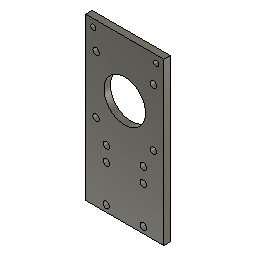
Carriage Plate P3 Printer (Autodesk Fusion 360 design; units mm, degrees)
Autodesk Fusion 360 part; units mm, degrees
sketch "Sketch1" plane through (0, 0, 0) normal (0, 1, 0) x (1, 0, 0)
  line L0 (32, 30) -> (-32, 30)
  line L1 (-32, 30) -> (-32, -30)
  line L2 (-32, -30) -> (32, -30)
  line L3 (32, -30) -> (32, 30)
  line L4 (32, 30) -> (-32, -30) construction
  line L5 (-32, 30) -> (32, -30) construction
  line L6 (-10, 2.5) -> (10, 2.5) construction
  line L7 (10, 2.5) -> (10, 22.5) construction
  line L8 (10, 22.5) -> (-10, 22.5) construction
  line L9 (-10, 22.5) -> (-10, 2.5) construction
  circle A0 centre (-10, 2.5) radius 1.75
  circle A1 centre (10, 2.5) radius 1.75
  circle A2 centre (10, 22.5) radius 1.75
  circle A3 centre (-10, 22.5) radius 1.75
  line L10 (28, 26) -> (-28, 26)
  line L11 (-28, 26) -> (-28, -26)
  line L12 (-28, -26) -> (28, -26)
  line L13 (28, -26) -> (28, 26)
  line L14 (-28, -26) -> (-24, -26)
  line L15 (-24, -26) -> (-24, 0)
  line L16 (-24, 0) -> (-28, 0)
  line L17 (-28, 0) -> (-28, -26)
  line L18 (28, -26) -> (24, -26)
  line L19 (24, -26) -> (24, 0)
  line L20 (24, 0) -> (28, 0)
  line L21 (28, 0) -> (28, -26)
  line L22 (21.15, -30) -> (-21.15, -30) construction
  line L23 (-21.15, -30) -> (-21.15, -22) construction
  line L24 (21.15, -22) -> (21.15, -30) construction
  line L25 (-21.15, -30) -> (21.15, -30)
  line L26 (21.15, -30) -> (21.15, -10)
  line L27 (21.15, -10) -> (-21.15, -10)
  line L28 (-21.15, -10) -> (-21.15, -30)
  line L29 (21.15, -10) -> (-21.15, -10)
  line L30 (-21.15, -10) -> (-21.15, -52.3)
  line L31 (-21.15, -52.3) -> (21.15, -52.3)
  line L32 (21.15, -52.3) -> (21.15, -10)
  line L33 (21.15, -52.3) -> (-21.15, -10) construction
  line L34 (-21.15, -52.3) -> (21.15, -10) construction
  line L35 (-15.5, -15.65) -> (15.5, -15.65) construction
  line L36 (15.5, -15.65) -> (15.5, -46.65) construction
  line L37 (15.5, -46.65) -> (-15.5, -46.65) construction
  line L38 (-15.5, -46.65) -> (-15.5, -15.65) construction
  line L39 (-15.5, -15.65) -> (15.5, -46.65) construction
  line L40 (15.5, -15.65) -> (-15.5, -46.65) construction
  circle A4 centre (15.5, -46.65) radius 1.75
  circle A5 centre (-15.5, -46.65) radius 1.75
  circle A6 centre (-15.5, -15.65) radius 1.75
  circle A7 centre (15.5, -15.65) radius 1.75
  circle A8 centre (0, -31.15) radius 11.25
  line L41 (-21.15, -26) -> (21.15, -26)
  line L42 (21.15, -26) -> (21.15, 26)
  line L43 (21.15, 26) -> (-21.15, 26)
  line L44 (-21.15, 26) -> (-21.15, -26)
  line L45 (21.15, 26) -> (-21.15, 26)
  line L46 (-21.15, 26) -> (-21.15, -1)
  line L47 (-21.15, -1) -> (21.15, -1)
  line L48 (21.15, -1) -> (21.15, 26)
  line L49 (21.15, -1) -> (-21.15, -1) construction
  line L50 (-21.15, -1) -> (-21.15, -10) construction
  line L51 (-21.15, -10) -> (21.15, -10) construction
  line L52 (21.15, -10) -> (21.15, -1) construction
  circle A9 centre (-10, -5.5) radius 1.75
  circle A10 centre (10, -5.5) radius 1.75
  line L53 (21.15, -52.3) -> (-21.15, -52.3)
  line L54 (-21.15, -52.3) -> (-21.15, -61.3)
  line L55 (-21.15, -61.3) -> (21.15, -61.3)
  line L56 (21.15, -61.3) -> (21.15, -52.3)
  circle A11 centre (-17, -57.2801) radius 1.4
  circle A12 centre (17, -57.3) radius 1.4
  point P0 (0, -26)
  point P1 (0, -31.15)
  dimension "d1" = 64
  dimension "d2" = 60
  dimension "d3" = 20
  dimension "d4" = 20
  dimension "d6" = 22
  dimension "d7" = 3.5
  dimension "d8" = 3.5
  dimension "d9" = 3.5
  dimension "d10" = 3.5
  dimension "d11" = -4
  dimension "d12" = 4
  dimension "d13" = 4
  dimension "d40" = 3.5
  dimension "d41" = 26
  dimension "d42" = 26
  dimension "d43" = 42.3
  dimension "d44" = 8
  dimension "d45" = 20
  dimension "d46" = 42.3
  dimension "d49" = 31
  dimension "d50" = 31
  dimension "d51" = 3.5
  dimension "d52" = 3.5
  dimension "d53" = 3.5
  dimension "d54" = 3.5
  dimension "d57" = 22.5
  dimension "d58" = 27
  dimension "d59" = 3.5
  dimension "d60" = 3.5
  dimension "d61" = 4.5
  dimension "d62" = 4.5
  dimension "d64" = 11.15
  dimension "d65" = 11.15
  dimension "d66" = 9
  dimension "d67" = 2.8
  dimension "d68" = 2.8
  dimension "d69" = 4
  dimension "d72" = 42.3
  dimension "d74" = 4.15
  dimension "d75" = 34
  constraint perpendicular L0 L1
  constraint parallel L0 L2
  constraint parallel L1 L3
  constraint horizontal L0
  constraint coincident L4 origin
  constraint coincident L5 origin
  constraint horizontal L6
  constraint vertical L7
  constraint horizontal L8
  constraint vertical L9
  constraint coincident L6.start L9.end
  constraint coincident L6.end L7.start
  constraint coincident L7.end L8.start
  constraint coincident L8.end L9.start
  constraint horizontal L14
  constraint vertical L15
  constraint horizontal L16
  constraint vertical L17
  constraint horizontal L18
  constraint vertical L19
  constraint horizontal L20
  constraint vertical L21
  constraint perpendicular L22 L23
  constraint parallel L23 L24
  constraint horizontal L22
  constraint midpoint L12 P0
  constraint horizontal L25
  constraint vertical L26
  constraint horizontal L27
  constraint vertical L28
  constraint horizontal L29
  constraint vertical L30
  constraint horizontal L31
  constraint vertical L32
  constraint perpendicular L33 L34
  constraint perpendicular L35 L36
  constraint parallel L35 L37
  constraint parallel L36 L38
  constraint horizontal L35
  constraint coincident L39 P1
  constraint coincident L40 P1
  constraint midpoint L33 P1
  constraint coincident L36.end L37.start
  constraint coincident L37.end L38.start
  constraint coincident L35.start L38.end
  constraint coincident L35.end L36.start
  constraint coincident P1 A8.centre
  constraint horizontal L41
  constraint vertical L42
  constraint horizontal L43
  constraint vertical L44
  constraint coincident L10 L42.end
  constraint midpoint L23 L41.start
  constraint horizontal L45
  constraint vertical L46
  constraint horizontal L47
  constraint vertical L48
  constraint horizontal L49
  constraint vertical L50
  constraint horizontal L51
  constraint vertical L52
  constraint horizontal L53
  constraint vertical L54
  constraint horizontal L55
  constraint vertical L56
  measures "d1" distance of L1.end L2.end L0.end
  measures "d2" distance of L0.end L1.end
  measures "d3" distance of L6.start L6.end
  measures "d4" distance of L6.start L8.end
  measures "d6" distance of L1 L9
  measures "d7" diameter of A0
  measures "d8" diameter of A1
  measures "d9" diameter of A2
  measures "d10" diameter of A3
  measures "d12" distance of L11.end L14.end
  measures "d13" distance of L12.end L18.end
  measures "d40" distance of L7.end L10
  measures "d41" distance of L14 L16
  measures "d42" distance of L18 L20
  measures "d43" distance of L23.end L24.start L0.end
  measures "d44" distance of L22.end L23.end L0.end
  measures "d45" distance of L22.end L27.end
  measures "d46" distance of L26.end L31.end
  measures "d49" distance of L36.end L37.end
  measures "d50" distance of L35.end L36.end
  measures "d51" diameter of A4
  measures "d52" diameter of A5
  measures "d53" diameter of A6
  measures "d54" diameter of A7
  measures "d57" diameter of A8
  measures "d58" distance of L42.end L47.end
  measures "d59" diameter of A9
  measures "d60" diameter of A10
  measures "d61" distance of L47 A10.centre
  measures "d62" distance of L47 A9.centre
  measures "d64" distance of L50 A9.centre
  measures "d65" distance of L52 A10.centre
  measures "d66" distance of L31.end L55.end
  measures "d67" diameter of A11
  measures "d68" diameter of A12
  measures "d69" distance of L55 A12.centre
  measures "d72" distance of L54 L56
  measures "d74" distance of L56 A12.centre
  measures "d75" horizontal distance of A11.centre A12.centre
extrude "Extrude1" add sketch "Sketch1" against normal blind 3.5 contours L27 L29 L42 L44 L47 | L10 L42 L43 L44 L45 L46 L47 L48
extrude "Extrude8" add sketch "Sketch1" against normal blind 3.5 contours L2 L25 L30 L31 L32 A8 L53 | L2 L12 L25 L26 L32 A8 L41 | L2 L12 L25 L28 L30 A8 L41 | L12 L26 L27 L28 L29 L30 L32 A8 L41 L42 L44 | L31 L53 L54 L55 L56
